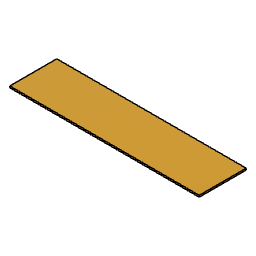
SB-frontPack v1 (Autodesk Fusion 360 design; units mm, degrees)
Autodesk Fusion 360 part; units mm, degrees
sketch "Sketch1" plane through (0, 0, 0) normal (0, 0, 1) x (1, 0, 0)
  line L0 (172.9, -42.9) -> (-172.9, -42.9)
  line L1 (-172.9, -42.9) -> (-172.9, 42.9)
  line L2 (-172.9, 42.9) -> (172.9, 42.9)
  line L3 (172.9, 42.9) -> (172.9, -42.9)
  line L4 (172.9, -42.9) -> (-172.9, 42.9) construction
  line L5 (-172.9, -42.9) -> (172.9, 42.9) construction
  dimension "d1" = 345.8
  dimension "d2" = 85.8
  constraint horizontal L0
  constraint perpendicular L0 L1
  constraint parallel L0 L2
  constraint parallel L1 L3
  constraint coincident L4 origin
  constraint coincident L5 origin
  measures "d1" distance of L1.end L2.end
  measures "d2" distance of L0.end L1.end
extrude "Extrude1" add sketch "Sketch1" along normal blind 2.9 makes body 1
copy_body "Body->Comp1" bodies 1 removing the originals makes body 2 in component "Dhakna"
component "Dhakna" placed x (1, 0, 0) y (0, 1, 0) z (0, 0, 1) at (0, 0, 0)
